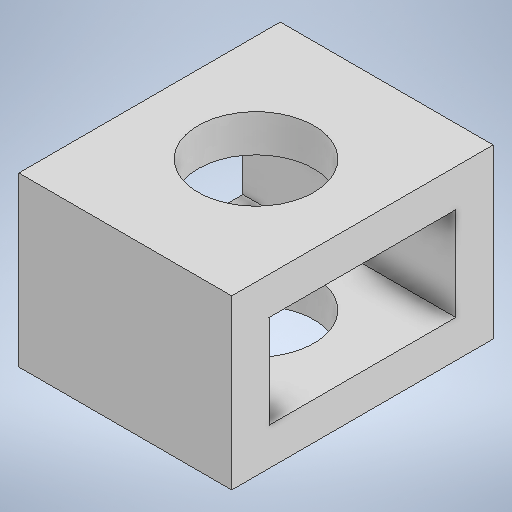
# Autodesk Inventor part: Part1
Saved by Autodesk Inventor 2025 (Build 290162000, 162)
## iProperties
Created: 2025-01-30
Part Number: Part1
Material: Generic
Document SubType Name: Modeling
Designer: 7008661
Density: 1 g/cm^3
Appearance: Default
Author: 7008661
Autodesk Inventor part; units mm, degrees
ref_plane "YZ Plane" through (0, 0, 0) normal (1, 0, 0) x (0, 1, 0)
ref_plane "XZ Plane" through (0, 0, 0) normal (0, 1, 0) x (-1, 0, 0)
ref_plane "XY Plane" through (0, 0, 0) normal (0, 0, 1) x (1, 0, 0)
sketch "Sketch2" plane through (0, 0, 0) normal (0, 1, 0) x (-1, 0, 0)
  line L0 (-5.7, 5) -> (5.7, 5)
  line L1 (5.7, 5) -> (5.7, -5)
  line L2 (5.7, -5) -> (-5.7, -5)
  line L3 (-5.7, -5) -> (-5.7, 5)
  line L4 (-5.7, 5) -> (5.7, -5) construction
  line L5 (5.7, 5) -> (-5.7, -5) construction
  circle A0 centre (0, 0) radius 2.6
  dimension "d0" = 11.4
  dimension "d1" = 10
  dimension "d2" = 5.2
  constraints: 12 end point, 2 midpoint, 2 parallel, 1 centre point, 1 coincident, 1 horizontal, 1 perpendicular
  measures "d0" distance of L1.end L2.end
  measures "d1" distance of L0.end L1.end
  measures "d2" diameter of A0
extrude "Extrusion1" add sketch "Sketch2" along normal blind 9
sketch "Sketch3" plane through (5.7, 0, -5) normal (0, 0, -1) x (-1, 0, 0)
  line L0 (0, 9) -> (11.4, 9) projected
  line L1 (0, 9) -> (0, 7)
  line L2 (0, 0) -> (0, 9) projected
  line L3 (0, 0) -> (0, 2)
  line L4 (0, 7) -> (0, 2)
  line L5 (0, 2) -> (11.4, 2)
  line L6 (11.4, 2) -> (11.4, 7)
  line L7 (11.4, 7) -> (0, 7)
  point P0 (5.7, 0)
  dimension "d5" = 2
  dimension "d6" = 2
  constraints: 12 end point, 2 parallel, 2 point on line, 1 collinear, 1 perpendicular
  measures "d5" distance of L0.start L1.end
  measures "d6" distance of L2.start L3.end
extrude "Extrusion2" cut sketch "Sketch3" against normal blind 10.5875
sketch "Sketch4" plane through (0, 0, 0) normal (0, -1, 0) x (1, 0, 0)
  line L0 (-5.7, -5) -> (-5.7, 5) projected
  line L1 (-5.7, 5) -> (-5.7, 7)
  line L2 (-5.7, 7) -> (5.7, 7)
  line L3 (5.7, 7) -> (5.7, -7)
  line L4 (5.7, -7) -> (-5.7, -7)
  line L5 (-5.7, -7) -> (-5.7, 7)
  line L6 (-5.7, 7) -> (-5.7, -7)
  line L7 (-5.7, -7) -> (-7.7, -7)
  line L8 (-7.7, -7) -> (-7.7, 7)
  line L9 (-7.7, 7) -> (-5.7, 7)
  line L10 (5.7, -7) -> (5.7, -5)
  line L11 (5.7, -5) -> (-5.7, -5)
  line L12 (-5.7, -5) -> (-5.7, -7)
  line L13 (-5.7, -7) -> (5.7, -7)
  line L14 (-5.7, 5) -> (-5.7, 7)
  line L15 (-5.7, 7) -> (5.7, 7)
  line L16 (5.7, 7) -> (5.7, 5)
  line L17 (5.7, 5) -> (-5.7, 5)
  line L18 (-5.7, -5) -> (-5.7, 5)
  line L19 (5.7, -5) -> (5.7, 5)
  point P0 (0, 0)
  dimension "d9" = 2
  dimension "d10" = 11.4
  dimension "d11" = 14
  dimension "d12" = 2
  constraints: 38 end point, 8 parallel, 5 perpendicular, 3 collinear, 1 horizontal, 1 point on line, 1 vertical
  measures "d9" distance of L0.end L1.end
  measures "d10" distance of L1.end L2.end
  measures "d11" distance of L2.end L3.end
  measures "d12" distance of L4.end L7.end
extrude "Extrusion3" add sketch "Sketch4" against normal up to surface (9 mm away) contours L11 L3 L4 L5 | L1 L2 L3 L17
sketch "Sketch6" plane through (0, 9, 0) normal (0, 1, 0) x (1, 0, 0)
  circle A0 centre (0, 0) radius 3.1
  dimension "d18" = 6.2
  constraints: 1 centre point, 1 coincident
  measures "d18" diameter of A0
extrude "Extrusion4" cut sketch "Sketch6" against normal blind 10
body "Solid1"
